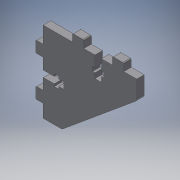
# Autodesk Inventor part: motor_brace_3
Saved by Autodesk Inventor 2019 (Build 230136000, 136)
## iProperties
Created: 2020-03-11
Part Number: motor_brace_3
Material: Generic
Document SubType Name: Modeling
Designer: Vijay
Density: 1 g/cm^3
Appearance: Default
Author: Vijay
Autodesk Inventor part; units mm, degrees
ref_plane "YZ Plane" through (0, 0, 0) normal (1, 0, 0) x (0, 1, 0)
ref_plane "XZ Plane" through (0, 0, 0) normal (0, 1, 0) x (-1, 0, 0)
ref_plane "XY Plane" through (0, 0, 0) normal (0, 0, 1) x (1, 0, 0)
sketch "Sketch1" plane through (0, 0, 0) normal (0, 0, 1) x (1, 0, 0)
  line L0 (0, -42.8392) -> (0, 0.8108) projected
  line L1 (0, 0) -> (49.5875, 0)
  line L2 (0, -42.8392) -> (10, -42.8392)
  line L3 (10, -42.8392) -> (49.5875, -10)
  line L4 (49.5875, -10) -> (49.5875, 0)
  line L5 (0, -42.8392) -> (0, 0)
  line L6 (0, 0) -> (49.5875, 0)
  line L7 (21.7117, 0) -> (36.5117, 0) construction
  dimension "d0" = 10
  dimension "d1" = 10
  constraints: 12 end point, 3 collinear, 1 horizontal, 1 parallel, 1 point on line, 1 other
  measures "d0" distance of L0.start L2.end
  measures "d1" distance of L3.end L1.end
extrude "Extrusion1" add sketch "Sketch1" against normal blind 4
fillet "Fillet1" radius 2 2 edges at (49.5875, -10, -2) (10, -42.8392, -2)
sketch "Sketch2" plane through (0, 0, 0) normal (0, 0, 1) x (1, 0, 0)
  line L0 (14.6536, -1.8875) -> (0, -1.8875) construction
  line L1 (0, -1.8875) -> (0, -8.7634) projected
  line L2 (0, -8.7634) -> (-6.35, -8.7634) projected
  line L3 (-6.35, -8.7634) -> (-6.35, -14.7634) projected
  line L4 (-6.35, -14.7634) -> (0, -14.7634) projected
  line L5 (0, -14.7634) -> (0, -20.8634) projected
  line L6 (0, -20.8634) -> (6, -20.8634) projected
  line L7 (6, -20.8634) -> (6, -19.6134) projected
  line L8 (6, -19.6134) -> (8, -19.6134) projected
  line L9 (8, -19.6134) -> (8, -20.8634) projected
  line L10 (8, -20.8634) -> (10.65, -20.8634) projected
  line L11 (10.65, -20.8634) -> (10.65, -23.8634) projected
  line L12 (10.65, -23.8634) -> (8, -23.8634) projected
  line L13 (8, -23.8634) -> (8, -25.1134) projected
  line L14 (8, -25.1134) -> (6, -25.1134) projected
  line L15 (6, -25.1134) -> (6, -23.8634) projected
  line L16 (6, -23.8634) -> (0, -23.8634) projected
  line L17 (0, -23.8634) -> (0, -29.9634) projected
  line L18 (0, -29.9634) -> (-6.35, -29.9634) projected
  line L19 (-6.35, -29.9634) -> (-6.35, -35.9634) projected
  line L20 (-6.35, -35.9634) -> (0, -35.9634) projected
  line L21 (0, -35.9634) -> (0, -42.8392) projected
  line L22 (0, -42.8392) -> (14.6536, -42.8392) projected
  line L23 (14.6536, -42.8392) -> (14.6536, -1.8875) construction
  line L24 (49.5875, -14.6536) -> (49.5875, 0) projected
  line L25 (49.5875, 0) -> (42.7117, 0) projected
  line L26 (42.7117, 0) -> (42.7117, 6.35) projected
  line L27 (42.7117, 6.35) -> (36.7117, 6.35) projected
  line L28 (36.7117, 6.35) -> (36.7117, 0) projected
  line L29 (36.7117, 0) -> (30.6117, 0) projected
  line L30 (30.6117, 0) -> (30.6117, -6) projected
  line L31 (30.6117, -6) -> (31.8617, -6) projected
  line L32 (31.8617, -6) -> (31.8617, -8) projected
  line L33 (31.8617, -8) -> (30.6117, -8) projected
  line L34 (30.6117, -8) -> (30.6117, -10.65) projected
  line L35 (30.6117, -10.65) -> (27.6117, -10.65) projected
  line L36 (27.6117, -10.65) -> (27.6117, -8) projected
  line L37 (27.6117, -8) -> (26.3617, -8) projected
  line L38 (26.3617, -8) -> (26.3617, -6) projected
  line L39 (26.3617, -6) -> (27.6117, -6) projected
  line L40 (27.6117, -6) -> (27.6117, 0) projected
  line L41 (27.6117, 0) -> (21.5117, 0) projected
  line L42 (21.5117, 0) -> (21.5117, 6.35) projected
  line L43 (21.5117, 6.35) -> (15.5117, 6.35) projected
  line L44 (15.5117, 6.35) -> (15.5117, 0) projected
  line L45 (15.5117, 0) -> (8.6359, 0) projected
  line L46 (8.6359, 0) -> (8.6359, -14.6536) construction
  line L47 (8.6359, -14.6536) -> (49.5875, -14.6536) construction
  line L48 (49.5875, 0) -> (0, -42.8392)
  line L49 (8.6359, 0) -> (0, -1.8875)
  point P0 (0, 0)
  constraints: 4 end point
extrude "Extrusion2" add sketch "Sketch2" against normal blind 4
sketch "Sketch3" plane through (0, 0, 0) normal (0, 0, 1) x (1, 0, 0)
  line L0 (14.6536, -1.8875) -> (0, -1.8875) projected
  line L1 (0, -1.8875) -> (0, -8.7634) projected
  line L2 (0, -8.7634) -> (-6.35, -8.7634) projected
  line L3 (-6.35, -8.7634) -> (-6.35, -14.7634) projected
  line L4 (-6.35, -14.7634) -> (0, -14.7634) projected
  line L5 (0, -14.7634) -> (0, -20.8634) projected
  line L6 (0, -20.8634) -> (6, -20.8634) projected
  line L7 (6, -20.8634) -> (6, -19.6134) projected
  line L8 (6, -19.6134) -> (8, -19.6134) projected
  line L9 (8, -19.6134) -> (8, -20.8634) projected
  line L10 (8, -20.8634) -> (10.65, -20.8634) projected
  line L11 (10.65, -20.8634) -> (10.65, -23.8634) projected
  line L12 (10.65, -23.8634) -> (8, -23.8634) projected
  line L13 (8, -23.8634) -> (8, -25.1134) projected
  line L14 (8, -25.1134) -> (6, -25.1134) projected
  line L15 (6, -25.1134) -> (6, -23.8634) projected
  line L16 (6, -23.8634) -> (0, -23.8634) projected
  line L17 (0, -23.8634) -> (0, -29.9634) projected
  line L18 (0, -29.9634) -> (-6.35, -29.9634) projected
  line L19 (-6.35, -29.9634) -> (-6.35, -35.9634) projected
  line L20 (-6.35, -35.9634) -> (0, -35.9634) projected
  line L21 (0, -35.9634) -> (0, -42.8392) projected
  line L22 (0, -42.8392) -> (14.6536, -42.8392) projected
  line L23 (14.6536, -42.8392) -> (14.6536, -1.8875) projected
  line L24 (49.5875, -14.6536) -> (49.5875, 0) projected
  line L25 (49.5875, 0) -> (42.7117, 0) projected
  line L26 (42.7117, 0) -> (42.7117, 6.35) projected
  line L27 (42.7117, 6.35) -> (36.7117, 6.35) projected
  line L28 (36.7117, 6.35) -> (36.7117, 0) projected
  line L29 (36.7117, 0) -> (30.6117, 0) projected
  line L30 (30.6117, 0) -> (30.6117, -6) projected
  line L31 (30.6117, -6) -> (31.8617, -6) projected
  line L32 (31.8617, -6) -> (31.8617, -8) projected
  line L33 (31.8617, -8) -> (30.6117, -8) projected
  line L34 (30.6117, -8) -> (30.6117, -10.65) projected
  line L35 (30.6117, -10.65) -> (27.6117, -10.65) projected
  line L36 (27.6117, -10.65) -> (27.6117, -8) projected
  line L37 (27.6117, -8) -> (26.3617, -8) projected
  line L38 (26.3617, -8) -> (26.3617, -6) projected
  line L39 (26.3617, -6) -> (27.6117, -6) projected
  line L40 (27.6117, -6) -> (27.6117, 0) projected
  line L41 (27.6117, 0) -> (21.5117, 0) projected
  line L42 (21.5117, 0) -> (21.5117, 6.35) projected
  line L43 (21.5117, 6.35) -> (15.5117, 6.35) projected
  line L44 (15.5117, 6.35) -> (15.5117, 0) projected
  line L45 (15.5117, 0) -> (8.6359, 0) projected
  line L46 (8.6359, 0) -> (8.6359, -14.6536) projected
  line L47 (8.6359, -14.6536) -> (49.5875, -14.6536) projected
  line L48 (0, -23.8634) -> (0, -20.8634)
  line L49 (0, -14.7634) -> (0, -29.9634) projected
  line L50 (27.6117, 0) -> (30.6117, 0)
  line L51 (36.7117, 0) -> (21.5117, 0) projected
  point P0 (0, 0)
  constraints: 4 end point, 1 collinear, 1 parallel
extrude "Extrusion3" cut sketch "Sketch3" against normal blind 4 contours L6 L7 L8 L9 L10 L11 L12 L13 L14 L15 L16 L48 | L50 L30 L31 L32 L33 L34 L35 L36 L37 L38 L39 L40
sketch "Sketch4" plane through (0, 0, 0) normal (0, 0, 1) x (1, 0, 0)
  line L0 (30.6117, 0) -> (30.6117, -6) projected
  line L1 (30.6117, -6) -> (31.8617, -6) projected
  line L2 (31.8617, -6) -> (31.8617, -8) projected
  line L3 (31.8617, -8) -> (30.6117, -8) projected
  line L4 (30.6117, -8) -> (30.6117, -10.65) projected
  line L5 (30.6117, -10.65) -> (27.6117, -10.65) projected
  line L6 (27.6117, -10.65) -> (27.6117, -8) projected
  line L7 (27.6117, -8) -> (26.3617, -8) projected
  line L8 (26.3617, -8) -> (26.3617, -6) projected
  line L9 (26.3617, -6) -> (27.6117, -6) projected
  line L10 (27.6117, -6) -> (27.6117, 0) projected
  line L11 (27.6117, 0) -> (21.5117, 0) projected
  line L12 (21.5117, 0) -> (21.5117, 6.35) projected
  line L13 (21.5117, 6.35) -> (15.5117, 6.35) projected
  line L14 (15.5117, 6.35) -> (15.5117, 0) projected
  line L15 (15.5117, 0) -> (0, 0) projected
  line L16 (0, 0) -> (0, -8.7634) projected
  line L17 (0, -8.7634) -> (-6.35, -8.7634) projected
  line L18 (-6.35, -8.7634) -> (-6.35, -14.7634) projected
  line L19 (-6.35, -14.7634) -> (0, -14.7634) projected
  line L20 (0, -14.7634) -> (0, -29.9634) projected
  line L21 (0, -29.9634) -> (-6.35, -29.9634) projected
  line L22 (-6.35, -29.9634) -> (-6.35, -35.9634) projected
  line L23 (-6.35, -35.9634) -> (0, -35.9634) projected
  line L24 (0, -35.9634) -> (0, -42.8392) projected
  line L25 (0, -42.8392) -> (9.2784, -42.8392) projected
  arc A0 (9.2784, -42.8392) -> (10.5554, -42.3785) centre (9.2784, -40.8392) ccw projected
  line L26 (10.5554, -42.3785) -> (48.8645, -10.5998) projected
  arc A1 (48.8645, -10.5998) -> (49.5875, -9.0605) centre (47.5875, -9.0605) ccw projected
  line L27 (49.5875, -9.0605) -> (49.5875, 0) projected
  line L28 (49.5875, 0) -> (42.7117, 0) projected
  line L29 (42.7117, 0) -> (42.7117, 6.35) projected
  line L30 (42.7117, 6.35) -> (36.7117, 6.35) projected
  line L31 (36.7117, 6.35) -> (36.7117, 0) projected
  line L32 (36.7117, 0) -> (30.6117, 0) projected
  line L33 (6, -23.8634) -> (0, -23.8634) projected
  line L34 (0, -23.8634) -> (0, -20.8634) projected
  line L35 (0, -20.8634) -> (6, -20.8634) projected
  line L36 (6, -20.8634) -> (6, -19.6134) projected
  line L37 (6, -19.6134) -> (8, -19.6134) projected
  line L38 (8, -19.6134) -> (8, -20.8634) projected
  line L39 (8, -20.8634) -> (10.65, -20.8634) projected
  line L40 (10.65, -20.8634) -> (10.65, -23.8634) projected
  line L41 (10.65, -23.8634) -> (8, -23.8634) projected
  line L42 (8, -23.8634) -> (8, -25.1134) projected
  line L43 (8, -25.1134) -> (6, -25.1134) projected
  line L44 (6, -25.1134) -> (6, -23.8634) projected
  line L45 (36.7117, 0) -> (30.6117, 0) projected
  line L46 (27.6117, 0) -> (30.6117, 0)
  line L47 (36.9117, 0) -> (36.9117, 6.15)
  line L48 (36.9117, 6.15) -> (42.5117, 6.15)
  line L49 (42.5117, 6.15) -> (42.5117, -0.2)
  line L50 (42.5117, -0.2) -> (49.3875, -0.2)
  line L51 (49.3875, -0.2) -> (49.3875, -9.0605)
  arc A2 (48.7368, -10.4459) -> (49.3875, -9.0605) centre (47.5875, -9.0605) ccw
  line L52 (48.7368, -10.4459) -> (10.4277, -42.2246)
  arc A3 (9.2784, -42.6392) -> (10.4277, -42.2246) centre (9.2784, -40.8392) ccw
  line L53 (9.2784, -42.6392) -> (0.2, -42.6392)
  line L54 (0.2, -42.6392) -> (0.2, -35.7634)
  line L55 (0.2, -35.7634) -> (-6.15, -35.7634)
  line L56 (-6.15, -35.7634) -> (-6.15, -30.1634)
  line L57 (-6.15, -30.1634) -> (0.2, -30.1634)
  line L58 (0.2, -30.1634) -> (0.2, -14.5634)
  line L59 (0.2, -14.5634) -> (-6.15, -14.5634)
  line L60 (-6.15, -14.5634) -> (-6.15, -8.9634)
  line L61 (-6.15, -8.9634) -> (0.2, -8.9634)
  line L62 (0.2, -8.9634) -> (0.2, -0.2)
  line L63 (0.2, -0.2) -> (15.7117, -0.2)
  line L64 (15.7117, -0.2) -> (15.7117, 6.15)
  line L65 (15.7117, 6.15) -> (21.3117, 6.15)
  line L66 (21.3117, 6.15) -> (21.3117, -0.2)
  line L67 (27.4117, -0.2) -> (27.4117, -5.8)
  line L68 (27.4117, -5.8) -> (26.1617, -5.8)
  line L69 (26.1617, -5.8) -> (26.1617, -8.2)
  line L70 (26.1617, -8.2) -> (27.4117, -8.2)
  line L71 (27.4117, -8.2) -> (27.4117, -10.85)
  line L72 (27.4117, -10.85) -> (30.8117, -10.85)
  line L73 (30.8117, -10.85) -> (30.8117, -8.2)
  line L74 (30.8117, -8.2) -> (32.0617, -8.2)
  line L75 (32.0617, -8.2) -> (32.0617, -5.8)
  line L76 (32.0617, -5.8) -> (30.8117, -5.8)
  line L77 (30.8117, -5.8) -> (30.8117, 0)
  line L78 (10.85, -20.6634) -> (8.2, -20.6634)
  line L79 (8.2, -20.6634) -> (8.2, -19.4134)
  line L80 (8.2, -19.4134) -> (5.8, -19.4134)
  line L81 (5.8, -19.4134) -> (5.8, -20.6634)
  line L82 (5.8, -20.6634) -> (-0.2, -20.6634)
  line L83 (-0.2, -20.6634) -> (-0.2, -24.0634)
  line L84 (-0.2, -24.0634) -> (5.8, -24.0634)
  line L85 (5.8, -24.0634) -> (5.8, -25.3134)
  line L86 (5.8, -25.3134) -> (8.2, -25.3134)
  line L87 (8.2, -25.3134) -> (8.2, -24.0634)
  line L88 (8.2, -24.0634) -> (10.85, -24.0634)
  line L89 (10.85, -24.0634) -> (10.85, -20.6634)
  line L90 (30.8117, -0.2) -> (30.8117, 0)
  line L91 (30.8117, 0) -> (27.4117, 0)
  line L92 (27.4117, 0) -> (27.4117, -0.2)
  point P0 (0, 0)
  dimension "d9" = 0.2
  dimension "d10" = 0.2
  constraints: 94 end point, 4 point on circle, 2 centre point, 1 horizontal, 1 parallel, 42 other
  measures "d9" distance between parallel lines of L10 L67
  measures "d10" distance between parallel lines of L39 L78
extrude "Extrusion4" cut sketch "Sketch4" against normal blind 25.4 contours L32 L77 L76 L75 L74 L73 L72 L71 L70 L69 L68 L67 L92 L11 L10 L9 L8 L7 L6 L5 L4 L3 L2 L1 L0 | L0 L1 L2 L3 L4 L5 L6 L7 L8 L9 L10 L46 | L82 L58 L35 L20 | L20 L84 L83 L82 | L35 L58 L33 L20 | L82 L81 L80 L79 L78 L89 L88 L87 L86 L85 L84 L58 L33 L44 L43 L42 L41 L40 L39 L38 L37 L36 L35 | L33 L58 L84 L20 | L35 L36 L37 L38 L39 L40 L41 L42 L43 L44 L33 L58
sketch "Sketch5" plane through (0, 0, 0) normal (0, 0, 1) x (1, 0, 0)
  line L0 (42.9117, 4) -> (46.4125, 4)
  line L1 (-4, -102.5091) -> (-4, 2)
  line L2 (61.4276, 22.986) -> (8.4509, 22.986)
  line L3 (8.4509, 22.986) -> (8.4509, 4)
  line L4 (8.4509, 4) -> (61.4276, 4)
  line L5 (61.4276, 4) -> (61.4276, 22.986)
  line L6 (-4, 2) -> (-14.2218, 2)
  line L7 (-14.2218, 2) -> (-14.2218, -39.6128)
  line L8 (-14.2218, -39.6128) -> (-4, -39.6128)
  line L9 (-4, -39.6128) -> (-4, 2)
  point P0 (0, 0)
  constraints: 20 end point, 4 parallel, 3 horizontal, 2 perpendicular, 1 vertical, 4 other
extrude "Extrusion5" cut sketch "Sketch5" against normal blind 25.4
fillet "Fillet2" radius 0.5 8 edges at (42.7117, 4, -2) (36.7117, 4, -2) (21.5117, 4, -2) (15.5117, 4, -2) (-4, -8.7634, -2) (-4, -14.7634, -2) (-4, -29.9634, -2) (-4, -35.9634, -2)
body "Solid1"
